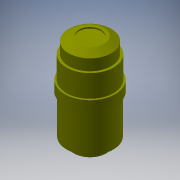
# Autodesk Inventor part: olympusXLSLPLN25XGMP_vFIN
Saved by Autodesk Inventor 2016 (Build 200138000, 138)
## iProperties
Created: 2015-08-12
Part Number: olympusXLSLPLN25XGMP_vFIN
Material: Generic
Document SubType Name: Modeling
Designer: CAIC
Density: 1 g/cm^3
Appearance: Default
Author: CAIC
Autodesk Inventor part; units mm, degrees
ref_plane "YZ Plane" through (0, 0, 0) normal (1, 0, 0) x (0, 1, 0)
ref_plane "XZ Plane" through (0, 0, 0) normal (0, 1, 0) x (-1, 0, 0)
sketch "Sketch1" plane through (0, 0, 0) normal (0, 0, 1) x (1, 0, 0)
  circle A0 centre (0, 0) radius 12.5
  dimension "d0" = 25
  constraints: 1 centre point, 1 coincident
  measures "d0" diameter of A0
extrude "Extrusion1" add sketch "Sketch1" along normal blind 5.3
sketch "Sketch2" plane through (0, 0, 5.3) normal (0, 0, 1) x (1, 0, 0)
  circle A0 centre (0, 0) radius 18
  dimension "d3" = 36
  constraints: 1 centre point, 1 coincident
  measures "d3" diameter of A0
extrude "Extrusion2" add sketch "Sketch2" along normal blind 29.8
sketch "Sketch3" plane through (0, 0, 35.1) normal (0, 0, 1) x (1, 0, 0)
  circle A0 centre (0, 0) radius 19.5
  dimension "d6" = 39
  constraints: 1 centre point, 1 coincident
  measures "d6" diameter of A0
extrude "Extrusion3" add sketch "Sketch3" along normal blind 8
sketch "Sketch4" plane through (0, 0, 43.1) normal (0, 0, 1) x (1, 0, 0)
  circle A0 centre (0, 0) radius 18.2
  dimension "d9" = 36.4
  constraints: 1 centre point, 1 coincident
  measures "d9" diameter of A0
extrude "Extrusion4" add sketch "Sketch4" along normal blind 17.2
sketch "Sketch5" plane through (0, 0, 60.3) normal (0, 0, 1) x (1, 0, 0)
  circle A0 centre (0, 0) radius 16.45
  dimension "d12" = 32.9
  constraints: 1 centre point, 1 coincident
  measures "d12" diameter of A0
extrude "Extrusion5" add sketch "Sketch5" along normal blind 1.8
sketch "Sketch6" plane through (0, 0, 62.1) normal (0, 0, 1) x (1, 0, 0)
  circle A0 centre (0, 0) radius 16.45
  dimension "d15" = 32.9
  constraints: 1 centre point, 1 coincident
  measures "d15" diameter of A0
extrude "Extrusion6" add sketch "Sketch6" along normal blind 6.8
sketch "Sketch7" plane through (0, 0, 68.9) normal (0, 0, 1) x (1, 0, 0)
  circle A0 centre (0, 0) radius 16.45
  dimension "d18" = 32.9
  constraints: 1 centre point, 1 coincident
  measures "d18" diameter of A0
ref_plane "Work Plane1" through (0, 0, 72.3) normal (0, 0, 1) x (1, 0, 0)
sketch "Sketch8" plane through (0, 0, 72.3) normal (0, 0, 1) x (1, 0, 0)
  circle A0 centre (0, 0) radius 10.75
  dimension "d20" = 21.5
  constraints: 1 centre point, 1 coincident
  measures "d20" diameter of A0
loft "Loft1" add profiles "Sketch8" section 1 edges at (-16.45, 0, 68.9)
sketch "Sketch9" plane through (0, 0, 72.3) normal (0, 0, 1) x (1, 0, 0)
  circle A0 centre (0, 0) radius 8.45
  dimension "d25" = 16.9
  constraints: 1 centre point, 1 coincident
  measures "d25" diameter of A0
extrude "Extrusion7" cut sketch "Sketch9" against normal blind 1
body "Solid1"
